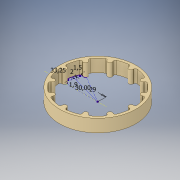
# Autodesk Inventor part: Enclosure
Saved by Autodesk Inventor 2018.3 (Build 223284000, 284)
## iProperties
Created: 2018-07-20
Part Number: Enclosure
Material: Generisch
Document SubType Name: Modeling
Designer: JochenAlt
Density: 1 g/cm^3
Appearance: Weizen
Author: JochenAlt
Autodesk Inventor part; units mm, degrees
ref_plane "YZ Plane" through (0, 0, 0) normal (1, 0, 0) x (0, 1, 0)
ref_plane "XZ Plane" through (0, 0, 0) normal (0, 1, 0) x (-1, 0, 0)
ref_plane "XY Plane" through (0, 0, 0) normal (0, 0, 1) x (1, 0, 0)
sketch "Skizze1" plane through (0, 0, 0) normal (0, 0, 1) x (1, 0, 0)
  line L0 (-46.7955, 0) -> (7.7993, 0) construction
  arc A0 (-28.7953, 16.625) -> (-33.25, 0) centre (0, 0) ccw
  arc A1 (-27.1, 0) -> (-28.8755, 1.8959) centre (-29, 0) ccw
  line L1 (0, 0) -> (-38.9963, 22.5145) construction
  line L2 (-29, 0) -> (0, 0) construction
  arc A2 (-25.9549, 12.7958) -> (-23.4693, 13.55) centre (-25.1147, 14.5) ccw
  arc A3 (-28.5207, 5.2509) -> (-29, 0) centre (0, 0) ccw construction
  arc A4 (-25.1147, 14.5) -> (-28.5207, 5.2509) centre (0, 0) ccw construction
  line L3 (-37.9513, 10.169) -> (0, 0) construction
  line L4 (-23.4693, 13.55) -> (-28.7953, 16.625)
  line L5 (-27.1, 0) -> (-33.25, 0)
  line L6 (-25.9549, 12.7958) -> (-26.425, 13.0276)
  line L7 (-28.8755, 1.8959) -> (-29.3985, 1.9303)
  arc A5 (-28.4657, 12.2762) -> (-30.7901, 3.6013) centre (0, 0) ccw
  arc A6 (-26.425, 13.0276) -> (-28.4657, 12.2762) centre (-27.0883, 11.6822) ccw
  arc A7 (-30.7901, 3.6013) -> (-29.3985, 1.9303) centre (-29.3003, 3.427) ccw
  point P0 (-28.0118, 7.5058)
  point P1 (-27.8046, 13.7078)
  point P2 (-30.9334, 2.031)
  dimension "d5" = 1.9
  dimension "d14" = 29
  dimension "d28" = 30
  dimension "d38" = 1.5
  dimension "d39" = 2
  dimension "d40" = 33.25
  constraints: 20 point on circle, 14 end point, 9 point on line, 8 centre point, 6 tangent, 3 coincident, 2 collinear, 2 equal radius, 1 other
  measures "d5" radius of A1
  measures "d14" distance of L1.start L2.start
  measures "d28" angle of L1 L0
  measures "d38" radius of A6
  measures "d39" radial gap between concentric circles of A5 A4
  measures "d40" radius of A0
extrude "Extrusion1" add sketch "Skizze1" along normal blind 11
pattern_circular "Runde Anordnung1" count 12 over 360 about axis through (0, 0, 0) along (0, 0, 1) of "Extrusion1"
